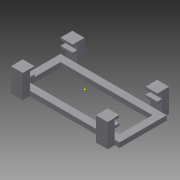
# Autodesk Inventor part: Ultrasound Sensor Holder
Saved by Autodesk Inventor 2015 (Build 190159000, 159)
## iProperties
Created: 2016-05-27
Part Number: Ultrasound Sensor Holder
Material: Generic
Document SubType Name: Modeling
Designer: Toby
Density: 1 g/cm^3
Appearance: Default
Author: Toby
Autodesk Inventor part; units mm, degrees
ref_plane "YZ Plane" through (0, 0, 0) normal (1, 0, 0) x (0, 1, 0)
ref_plane "XZ Plane" through (0, 0, 0) normal (0, 1, 0) x (-1, 0, 0)
ref_plane "XY Plane" through (0, 0, 0) normal (0, 0, 1) x (1, 0, 0)
sketch "Sketch1" plane through (0, 0, 0) normal (0, 0, 1) x (1, 0, 0)
  line L0 (-18.1542, 7.9766) -> (26.8458, 7.9766)
  line L1 (26.8458, 7.9766) -> (26.8458, -12.0234)
  line L2 (26.8458, -12.0234) -> (-18.1542, -12.0234)
  line L3 (-18.1542, -12.0234) -> (-18.1542, 7.9766)
  line L4 (-15.1542, 4.9766) -> (23.8458, 4.9766)
  line L5 (23.8458, 4.9766) -> (23.8458, -9.0234)
  line L6 (23.8458, -9.0234) -> (-15.1542, -9.0234)
  line L7 (-15.1542, -9.0234) -> (-15.1542, 4.9766)
  point P0 (0, 0)
  dimension "d0" = 45
  dimension "d1" = 20
  dimension "d2" = 3
  dimension "d3" = 3
  dimension "d4" = 3
  dimension "d5" = 3
  constraints: 16 end point, 4 parallel, 2 horizontal, 2 perpendicular
  measures "d0" distance of L0.start L0.end
  measures "d1" distance of L2.end L0.start
  measures "d2" distance between parallel lines of L4 L0
  measures "d3" distance between parallel lines of L2 L6
  measures "d4" distance between parallel lines of L3 L7
  measures "d5" distance between parallel lines of L1 L5
extrude "Extrusion1" add sketch "Sketch1" along normal blind 2
sketch "Sketch2" plane through (0, 0, 2) normal (0, 0, 1) x (1, 0, 0)
  point P0 (0, 0)
sketch "Sketch3" plane through (-18.1542, 7.9766, 0) normal (0, 1, 0) x (1, 0, 0)
  line L0 (3, -2) -> (42, -2) projected
  line L1 (2, 0) -> (7, 0)
  line L2 (7, 0) -> (7, -2)
  line L3 (7, -2) -> (2, -2)
  line L4 (2, -2) -> (2, 0)
  line L5 (42, 0) -> (3, 0) projected
  line L6 (45, -2) -> (0, -2) projected
  line L7 (38, 0) -> (43, 0)
  line L8 (43, 0) -> (43, -2)
  line L9 (43, -2) -> (38, -2)
  line L10 (38, -2) -> (38, 0)
  line L11 (0, 0) -> (0, -2) projected
  line L12 (45, 0) -> (45, -2) projected
  point P0 (18.1542, 0)
  dimension "d8" = 2
  dimension "d9" = 2
  dimension "d10" = 5
  dimension "d11" = 5
  constraints: 16 end point, 4 parallel, 3 point on line, 2 horizontal, 2 perpendicular
  measures "d8" distance between parallel lines of L11 L4
  measures "d9" distance between parallel lines of L12 L8
  measures "d10" distance of L1.start L1.end
  measures "d11" distance of L7.start L7.end
extrude "Extrusion2" add sketch "Sketch3" along normal blind 3 contours L3 L4 L1 L2 L0 | L10 L5 L7 L8 L6 L0
sketch "Sketch4" plane through (-18.1542, -12.0234, 0) normal (0, -1, 0) x (1, 0, 0)
  line L0 (45, 0) -> (0, 0) projected
  line L1 (2, 1.9967) -> (7, 1.9967)
  line L2 (7, 1.9967) -> (7, 0)
  line L3 (7, 0) -> (2, 0)
  line L4 (2, 0) -> (2, 1.9967)
  line L5 (43, 1.9967) -> (38, 1.9967)
  line L6 (38, 1.9967) -> (38, 0)
  line L7 (38, 0) -> (43, 0)
  line L8 (43, 0) -> (43, 1.9967)
  line L9 (45, 0) -> (45, 2) projected
  line L10 (0, 0) -> (0, 2) projected
  point P0 (18.1542, 0)
  dimension "d14" = 2
  dimension "d15" = 2
  dimension "d16" = 5
  dimension "d17" = 5
  constraints: 16 end point, 4 parallel, 2 horizontal, 2 perpendicular, 2 point on line
  measures "d14" distance between parallel lines of L9 L8
  measures "d15" distance between parallel lines of L10 L4
  measures "d16" distance of L1.start L1.end
  measures "d17" distance of L5.start L5.end
extrude "Extrusion3" add sketch "Sketch4" along normal blind 3
sketch "Sketch5" plane through (0, 0, 2) normal (0, 0, 1) x (1, 0, 0)
  point P0 (0, 0)
sketch "Sketch6" plane through (0, 0, 2) normal (0, 0, 1) x (1, 0, 0)
  line L0 (-16.1542, 10.9766) -> (-10.9816, 10.9766)
  line L1 (-10.9816, 10.9766) -> (-10.9816, 7.9766)
  line L2 (-10.9816, 7.9766) -> (-16.1542, 7.9766)
  line L3 (-16.1542, 7.9766) -> (-16.1542, 10.9766)
  line L4 (19.8458, 10.9766) -> (24.8959, 10.9766)
  line L5 (24.8959, 10.9766) -> (24.8959, 7.9766)
  line L6 (24.8959, 7.9766) -> (19.8458, 7.9766)
  line L7 (19.8458, 7.9766) -> (19.8458, 10.9766)
  line L8 (-18.1542, -12.0234) -> (26.8458, -12.0234) projected
  line L9 (-16.1542, -12.0234) -> (-11.1542, -12.0234)
  line L10 (-11.1542, -12.0234) -> (-11.1542, -15.0234)
  line L11 (-11.1542, -15.0234) -> (-16.1542, -15.0234)
  line L12 (-16.1542, -15.0234) -> (-16.1542, -12.0234)
  line L13 (19.8458, -12.0234) -> (24.8458, -12.0234)
  line L14 (24.8458, -12.0234) -> (24.8458, -15.0234)
  line L15 (24.8458, -15.0234) -> (19.8458, -15.0234)
  line L16 (19.8458, -15.0234) -> (19.8458, -12.0234)
  point P0 (0, 0)
  constraints: 32 end point, 8 parallel, 4 horizontal, 4 perpendicular, 3 point on line
extrude "Extrusion4" add sketch "Sketch6" along normal blind 8
sketch "Sketch7" plane through (-16.1542, -12.0234, 2) normal (0, 1, 0) x (1, 0, 0)
  line L0 (5, 0) -> (5, -8) projected
  line L1 (0, -8) -> (5, -8)
  line L2 (5, -8) -> (5, -7)
  line L3 (5, -7) -> (0, -7)
  line L4 (0, -7) -> (0, -8)
  line L5 (36, -8) -> (40.8353, -8)
  line L6 (40.8353, -8) -> (40.8353, -7)
  line L7 (40.8353, -7) -> (36, -7)
  line L8 (36, -7) -> (36, -8)
  point P0 (16.1542, 2)
  dimension "d22" = 1
  dimension "d23" = 1
  constraints: 16 end point, 4 parallel, 2 horizontal, 2 perpendicular, 2 point on line
  measures "d22" distance between parallel lines of L1 L3
  measures "d23" distance between parallel lines of L5 L7
extrude "Extrusion5" add sketch "Sketch7" along normal blind 2
sketch "Sketch8" plane through (-16.1542, -12.0234, 2) normal (0, 1, 0) x (1, 0, 0)
  line L0 (0, 0) -> (0, -8) projected
  line L1 (5, 0) -> (5, -8) projected
  line L2 (0, -4) -> (5, -4)
  line L3 (5, -4) -> (5, -5)
  line L4 (5, -5) -> (0, -5)
  line L5 (0, -5) -> (0, -4)
  line L6 (36.0707, -5) -> (40.8694, -5)
  line L7 (40.8694, -5) -> (40.8694, -4)
  line L8 (40.8694, -4) -> (36.0707, -4)
  line L9 (36.0707, -4) -> (36.0707, -5)
  line L10 (0, -7) -> (5, -7) projected
  point P0 (16.1542, 2)
  dimension "d26" = 1
  dimension "d27" = 2
  constraints: 16 end point, 4 parallel, 3 point on line, 2 horizontal, 2 perpendicular, 1 midpoint
  measures "d26" distance between parallel lines of L4 L2
  measures "d27" distance between parallel lines of L10 L4
extrude "Extrusion6" add sketch "Sketch8" along normal blind 2 contours L2 L1 L4 L0 | L9 L8 L7 L6
sketch "Sketch9" plane through (-16.1542, 7.9766, 2) normal (0, -1, 0) x (1, 0, 0)
  line L0 (5.1726, 0) -> (5.1726, 8) projected
  line L1 (0, 8) -> (5.1726, 8)
  line L2 (5.1726, 8) -> (5.1726, 7)
  line L3 (5.1726, 7) -> (0, 7)
  line L4 (0, 7) -> (0, 8)
  line L5 (0, 0) -> (0, 8) projected
  line L6 (0, 5) -> (5.1726, 5)
  line L7 (5.1726, 5) -> (5.1726, 4)
  line L8 (5.1726, 4) -> (0, 4)
  line L9 (0, 4) -> (0, 5)
  line L10 (36.1034, 8) -> (41.097, 8)
  line L11 (41.097, 8) -> (41.097, 7)
  line L12 (41.097, 7) -> (36.1034, 7)
  line L13 (36.1034, 7) -> (36.1034, 8)
  line L14 (36, 0) -> (36, 8) projected
  line L15 (41.0501, 0) -> (41.0501, 8) projected
  line L16 (36, 5) -> (41.0501, 5)
  line L17 (41.0501, 5) -> (41.0501, 4)
  line L18 (41.0501, 4) -> (36, 4)
  line L19 (36, 4) -> (36, 5)
  point P0 (16.1542, -2)
  dimension "d30" = 1
  dimension "d31" = 2
  dimension "d32" = 1
  constraints: 32 end point, 8 parallel, 7 point on line, 4 horizontal, 4 perpendicular, 2 midpoint
  measures "d30" distance between parallel lines of L1 L3
  measures "d31" distance between parallel lines of L6 L3
  measures "d32" distance between parallel lines of L8 L6
extrude "Extrusion7" add sketch "Sketch9" along normal blind 2 contours L8 L5 L6 L0 | L3 L4 L1 L0 | L15 L18 L14 L16 | L10 L15 L12 L13 | L10 L11 L12 L15
body "Solid1"
